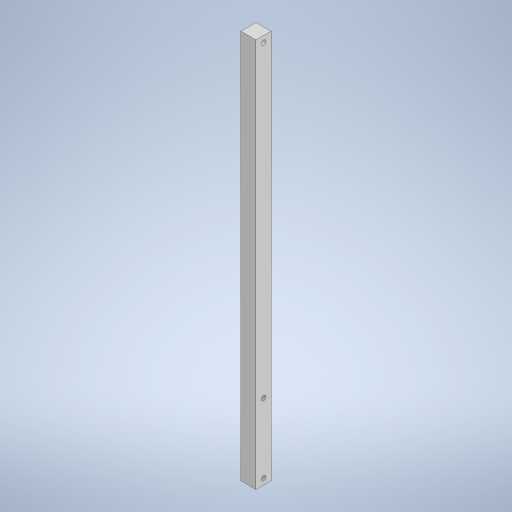
# Autodesk Inventor part: Naname
Saved by Autodesk Inventor 2023 (Build 270158000, 158)
## iProperties
Created: 2022-10-24
Part Number: Naname
Material: 一般
Document SubType Name: Modeling
Designer: banru
Density: 1 g/cm^3
Appearance: 既定
Author: banru
Autodesk Inventor part; units mm, degrees
ref_plane "YZ Plane" through (0, 0, 0) normal (1, 0, 0) x (0, 1, 0)
ref_plane "XZ Plane" through (0, 0, 0) normal (0, 1, 0) x (-1, 0, 0)
ref_plane "XY Plane" through (0, 0, 0) normal (0, 0, 1) x (1, 0, 0)
sketch "スケッチ1" plane through (0, 0, 0) normal (1, 0, 0) x (0, 1, 0)
  line L0 (0, 0) -> (258, 0)
  line L1 (258, 0) -> (258, -10)
  line L2 (258, -10) -> (0, -10)
  line L3 (0, -10) -> (0, 0)
  dimension "d0" = 258
  dimension "d1" = 10
  constraints: 8 end point, 2 parallel, 1 horizontal, 1 perpendicular
  measures "d0" distance of L1.end L2.end
  measures "d1" distance of L0.end L1.end
extrude "押し出し1" add sketch "スケッチ1" along normal blind 10
sketch "スケッチ2" plane through (10, 0, 0) normal (1, 0, 0) x (0, 0, -1)
  line L0 (0, 0) -> (10, 0) projected
  line L1 (10, 258) -> (0, 258) projected
  point P0 (5, 4)
  point P1 (5, 50)
  point P2 (5, 254)
  point P3 (5, 0)
  point P4 (5, 0)
  point P5 (5, 0)
  point P6 (5, 0)
  point P7 (5, 258)
  dimension "d4" = 4
  dimension "d5" = 50
  dimension "d6" = 4
  constraints: 5 midpoint, 3 vertical alignment
  measures "d4" distance of point (5, 0) point (5, 4)
  measures "d5" distance of point (5, 0) point (5, 50)
  measures "d6" distance of point (5, 258) point (5, 254)
hole "穴1" at (10, 4, -5) at (10, 50, -5) at (10, 254, -5) direction (-1, 0, 0) diameter 3.1 end through all
